Autodesk Fusion 360 part; units mm, degrees
note: some values were not read from the file. Set by a fixed rule: which face or edge a step refers to.
(part 2 of 4)
  spline S17 degree 5 poles (16.9837, -27.7093) (16.9833, -27.6954) (16.9825, -27.6677) (16.9812, -27.6262) (16.9792, -27.5708) (16.9764, -27.5018) (16.9734, -27.4329) (16.97, -27.364) (16.9664, -27.2952) (16.9624, -27.2266) (16.9582, -27.158) (16.9536, -27.0896) (16.9488, -27.0213) (16.9436, -26.953) (16.9381, -26.8849) (16.9323, -26.8169) (16.9262, -26.749) (16.9198, -26.6812) (16.9131, -26.6136) (16.906, -26.546) (16.8987, -26.4786) (16.891, -26.4113) (16.883, -26.3441) (16.8746, -26.2771) (16.866, -26.2101) (16.857, -26.1433) (16.8477, -26.0767) (16.838, -26.0102) (16.8281, -25.9438) (16.8178, -25.8775) (16.8071, -25.8114) (16.7961, -25.7455) (16.7848, -25.6797) (16.7731, -25.614) (16.761, -25.5485) (16.7486, -25.4831) (16.7359, -25.4179) (16.7228, -25.3529) (16.7093, -25.288) (16.6955, -25.2233) (16.6813, -25.1588) (16.6667, -25.0945) (16.6517, -25.0303) (16.6364, -24.9663) (16.6206, -24.9025) (16.6045, -24.8389) (16.5879, -24.7755) (16.571, -24.7123) (16.5537, -24.6492) (16.536, -24.5864) (16.5178, -24.5238) (16.4992, -24.4614) (16.4801, -24.3993) (16.4606, -24.3375) (16.4405, -24.2758) (16.4201, -24.2144) (16.3992, -24.1533) (16.3779, -24.0923) (16.3562, -24.0316) (16.3339, -23.9712) (16.3111, -23.9111) (16.2876, -23.8514) (16.2633, -23.7922) (16.2383, -23.7333) (16.2126, -23.6749) (16.1864, -23.6167) (16.1599, -23.5588) (16.1331, -23.501) (16.1057, -23.4436) (16.0774, -23.3868) (16.0476, -23.3309) (16.0221, -23.2873) (16.0018, -23.2552) (15.9877, -23.2342) (15.9805, -23.2237) knots -1 -1 -1 -1 -1 -1 -0.98571429 -0.97142857 -0.95714286 -0.94285714 -0.92857143 -0.91428571 -0.9 -0.88571429 -0.87142857 -0.85714286 -0.84285714 -0.82857143 -0.81428571 -0.8 -0.78571429 -0.77142857 -0.75714286 -0.74285714 -0.72857143 -0.71428571 -0.7 -0.68571429 -0.67142857 -0.65714286 -0.64285714 -0.62857143 -0.61428571 -0.6 -0.58571429 -0.57142857 -0.55714286 -0.54285714 -0.52857143 -0.51428571 -0.5 -0.48571429 -0.47142857 -0.45714286 -0.44285714 -0.42857143 -0.41428571 -0.4 -0.38571429 -0.37142857 -0.35714286 -0.34285714 -0.32857143 -0.31428571 -0.3 -0.28571429 -0.27142857 -0.25714286 -0.24285714 -0.22857143 -0.21428571 -0.2 -0.18571429 -0.17142857 -0.15714286 -0.14285714 -0.12857143 -0.11428571 -0.1 -0.08571429 -0.07142857 -0.05714286 -0.04285714 -0.02857143 -0.01428571 0 0 0 0 0 0
  line L17 (15.9805, -23.2237) -> (15.7785, -22.9298)
  arc A35 (15.9864, -21.6955) -> (15.7785, -22.9298) centre (16.5203, -22.42) ccw
  arc A36 (15.9864, -21.6955) -> (16.8187, -21.0569) centre (0, 0) ccw
  arc A37 (18.0647, -21.1755) -> (16.8187, -21.0569) centre (17.3803, -21.7601) ccw
  line L18 (18.0647, -21.1755) -> (18.2963, -21.4468)
  spline S18 degree 5 poles (18.2963, -21.4468) (18.3046, -21.4564) (18.3212, -21.4754) (18.3469, -21.5033) (18.3825, -21.5393) (18.4288, -21.5826) (18.4763, -21.6246) (18.5247, -21.6659) (18.5735, -21.7068) (18.6226, -21.7474) (18.6721, -21.7877) (18.7219, -21.8276) (18.7722, -21.867) (18.8232, -21.9058) (18.8747, -21.944) (18.9269, -21.9816) (18.9795, -22.0187) (19.0325, -22.0554) (19.0858, -22.0917) (19.1395, -22.1277) (19.1935, -22.1634) (19.2479, -22.1987) (19.3026, -22.2336) (19.3576, -22.2681) (19.413, -22.3022) (19.4688, -22.336) (19.5249, -22.3694) (19.5813, -22.4024) (19.638, -22.4351) (19.695, -22.4675) (19.7522, -22.4995) (19.8098, -22.5312) (19.8676, -22.5626) (19.9257, -22.5937) (19.9841, -22.6244) (20.0428, -22.6549) (20.1017, -22.685) (20.1609, -22.7148) (20.2203, -22.7443) (20.28, -22.7735) (20.3399, -22.8023) (20.4, -22.8309) (20.4604, -22.8592) (20.5211, -22.8872) (20.5819, -22.9149) (20.643, -22.9423) (20.7043, -22.9694) (20.7659, -22.9962) (20.8276, -23.0228) (20.8896, -23.049) (20.9518, -23.075) (21.0142, -23.1007) (21.0768, -23.1261) (21.1396, -23.1512) (21.2027, -23.176) (21.2659, -23.2006) (21.3293, -23.2249) (21.3929, -23.2489) (21.4567, -23.2726) (21.5207, -23.2961) (21.5849, -23.3193) (21.6493, -23.3422) (21.7139, -23.3649) (21.7786, -23.3872) (21.8436, -23.4094) (21.9087, -23.4312) (21.974, -23.4528) (22.0394, -23.4741) (22.1051, -23.4952) (22.1709, -23.516) (22.2369, -23.5365) (22.2898, -23.5527) (22.3295, -23.5648) (22.3561, -23.5727) (22.3694, -23.5767) knots 0 0 0 0 0 0 0.01428571 0.02857143 0.04285714 0.05714286 0.07142857 0.08571429 0.1 0.11428571 0.12857143 0.14285714 0.15714286 0.17142857 0.18571429 0.2 0.21428571 0.22857143 0.24285714 0.25714286 0.27142857 0.28571429 0.3 0.31428571 0.32857143 0.34285714 0.35714286 0.37142857 0.38571429 0.4 0.41428571 0.42857143 0.44285714 0.45714286 0.47142857 0.48571429 0.5 0.51428571 0.52857143 0.54285714 0.55714286 0.57142857 0.58571429 0.6 0.61428571 0.62857143 0.64285714 0.65714286 0.67142857 0.68571429 0.7 0.71428571 0.72857143 0.74285714 0.75714286 0.77142857 0.78571429 0.8 0.81428571 0.82857143 0.84285714 0.85714286 0.87142857 0.88571429 0.9 0.91428571 0.92857143 0.94285714 0.95714286 0.97142857 0.98571429 1 1 1 1 1 1
  arc A38 (22.3694, -23.5767) -> (23.5767, -22.3694) centre (0, 0) ccw
  spline S19 degree 5 poles (23.5767, -22.3694) (23.5727, -22.3561) (23.5648, -22.3295) (23.5527, -22.2898) (23.5365, -22.2369) (23.516, -22.1709) (23.4952, -22.1051) (23.4741, -22.0394) (23.4528, -21.974) (23.4312, -21.9087) (23.4094, -21.8436) (23.3872, -21.7786) (23.3649, -21.7139) (23.3422, -21.6493) (23.3193, -21.5849) (23.2961, -21.5207) (23.2726, -21.4567) (23.2489, -21.3929) (23.2249, -21.3293) (23.2006, -21.2659) (23.176, -21.2027) (23.1512, -21.1396) (23.1261, -21.0768) (23.1007, -21.0142) (23.075, -20.9518) (23.049, -20.8896) (23.0228, -20.8276) (22.9962, -20.7659) (22.9694, -20.7043) (22.9423, -20.643) (22.9149, -20.5819) (22.8872, -20.5211) (22.8592, -20.4604) (22.8309, -20.4) (22.8023, -20.3399) (22.7735, -20.28) (22.7443, -20.2203) (22.7148, -20.1609) (22.685, -20.1017) (22.6549, -20.0428) (22.6244, -19.9841) (22.5937, -19.9257) (22.5626, -19.8676) (22.5312, -19.8098) (22.4995, -19.7522) (22.4675, -19.695) (22.4351, -19.638) (22.4024, -19.5813) (22.3694, -19.5249) (22.336, -19.4688) (22.3022, -19.413) (22.2681, -19.3576) (22.2336, -19.3026) (22.1987, -19.2479) (22.1634, -19.1935) (22.1277, -19.1395) (22.0917, -19.0858) (22.0554, -19.0325) (22.0187, -18.9795) (21.9816, -18.9269) (21.944, -18.8747) (21.9058, -18.8232) (21.867, -18.7722) (21.8276, -18.7219) (21.7877, -18.6721) (21.7474, -18.6226) (21.7068, -18.5735) (21.6659, -18.5247) (21.6246, -18.4763) (21.5826, -18.4288) (21.5393, -18.3825) (21.5033, -18.3469) (21.4754, -18.3212) (21.4564, -18.3046) (21.4468, -18.2963) knots -1 -1 -1 -1 -1 -1 -0.98571429 -0.97142857 -0.95714286 -0.94285714 -0.92857143 -0.91428571 -0.9 -0.88571429 -0.87142857 -0.85714286 -0.84285714 -0.82857143 -0.81428571 -0.8 -0.78571429 -0.77142857 -0.75714286 -0.74285714 -0.72857143 -0.71428571 -0.7 -0.68571429 -0.67142857 -0.65714286 -0.64285714 -0.62857143 -0.61428571 -0.6 -0.58571429 -0.57142857 -0.55714286 -0.54285714 -0.52857143 -0.51428571 -0.5 -0.48571429 -0.47142857 -0.45714286 -0.44285714 -0.42857143 -0.41428571 -0.4 -0.38571429 -0.37142857 -0.35714286 -0.34285714 -0.32857143 -0.31428571 -0.3 -0.28571429 -0.27142857 -0.25714286 -0.24285714 -0.22857143 -0.21428571 -0.2 -0.18571429 -0.17142857 -0.15714286 -0.14285714 -0.12857143 -0.11428571 -0.1 -0.08571429 -0.07142857 -0.05714286 -0.04285714 -0.02857143 -0.01428571 0 0 0 0 0 0
  line L19 (21.4468, -18.2963) -> (21.1755, -18.0647)
  arc A39 (21.0569, -16.8187) -> (21.1755, -18.0647) centre (21.7601, -17.3803) ccw
  arc A40 (21.0569, -16.8187) -> (21.6955, -15.9864) centre (0, 0) ccw
  arc A41 (22.9298, -15.7785) -> (21.6955, -15.9864) centre (22.42, -16.5203) ccw
  line L20 (22.9298, -15.7785) -> (23.2237, -15.9805)
  spline S20 degree 5 poles (23.2237, -15.9805) (23.2342, -15.9877) (23.2552, -16.0018) (23.2873, -16.0221) (23.3309, -16.0476) (23.3868, -16.0774) (23.4436, -16.1057) (23.501, -16.1331) (23.5588, -16.1599) (23.6167, -16.1864) (23.6749, -16.2126) (23.7333, -16.2383) (23.7922, -16.2633) (23.8514, -16.2876) (23.9111, -16.3111) (23.9712, -16.3339) (24.0316, -16.3562) (24.0923, -16.3779) (24.1533, -16.3992) (24.2144, -16.4201) (24.2758, -16.4405) (24.3375, -16.4606) (24.3993, -16.4801) (24.4614, -16.4992) (24.5238, -16.5178) (24.5864, -16.536) (24.6492, -16.5537) (24.7123, -16.571) (24.7755, -16.5879) (24.8389, -16.6045) (24.9025, -16.6206) (24.9663, -16.6364) (25.0303, -16.6517) (25.0945, -16.6667) (25.1588, -16.6813) (25.2233, -16.6955) (25.288, -16.7093) (25.3529, -16.7228) (25.4179, -16.7359) (25.4831, -16.7486) (25.5485, -16.761) (25.614, -16.7731) (25.6797, -16.7848) (25.7455, -16.7961) (25.8114, -16.8071) (25.8775, -16.8178) (25.9438, -16.8281) (26.0102, -16.838) (26.0767, -16.8477) (26.1433, -16.857) (26.2101, -16.866) (26.2771, -16.8746) (26.3441, -16.883) (26.4113, -16.891) (26.4786, -16.8987) (26.546, -16.906) (26.6136, -16.9131) (26.6812, -16.9198) (26.749, -16.9262) (26.8169, -16.9323) (26.8849, -16.9381) (26.953, -16.9436) (27.0213, -16.9488) (27.0896, -16.9536) (27.158, -16.9582) (27.2266, -16.9624) (27.2952, -16.9664) (27.364, -16.97) (27.4329, -16.9734) (27.5018, -16.9764) (27.5708, -16.9792) (27.6262, -16.9812) (27.6677, -16.9825) (27.6954, -16.9833) (27.7093, -16.9837) knots 0 0 0 0 0 0 0.01428571 0.02857143 0.04285714 0.05714286 0.07142857 0.08571429 0.1 0.11428571 0.12857143 0.14285714 0.15714286 0.17142857 0.18571429 0.2 0.21428571 0.22857143 0.24285714 0.25714286 0.27142857 0.28571429 0.3 0.31428571 0.32857143 0.34285714 0.35714286 0.37142857 0.38571429 0.4 0.41428571 0.42857143 0.44285714 0.45714286 0.47142857 0.48571429 0.5 0.51428571 0.52857143 0.54285714 0.55714286 0.57142857 0.58571429 0.6 0.61428571 0.62857143 0.64285714 0.65714286 0.67142857 0.68571429 0.7 0.71428571 0.72857143 0.74285714 0.75714286 0.77142857 0.78571429 0.8 0.81428571 0.82857143 0.84285714 0.85714286 0.87142857 0.88571429 0.9 0.91428571 0.92857143 0.94285714 0.95714286 0.97142857 0.98571429 1 1 1 1 1 1
  arc A42 (27.7093, -16.9837) -> (28.563, -15.5051) centre (0, 0) ccw
  spline S21 degree 5 poles (28.563, -15.5051) (28.5557, -15.4933) (28.5411, -15.4697) (28.5192, -15.4344) (28.4898, -15.3875) (28.4529, -15.329) (28.4158, -15.2709) (28.3785, -15.2129) (28.3409, -15.1552) (28.3032, -15.0977) (28.2652, -15.0405) (28.2271, -14.9835) (28.1887, -14.9267) (28.1501, -14.8702) (28.1113, -14.814) (28.0723, -14.758) (28.033, -14.7022) (27.9936, -14.6467) (27.9539, -14.5915) (27.9141, -14.5365) (27.874, -14.4818) (27.8337, -14.4274) (27.7931, -14.3732) (27.7524, -14.3193) (27.7114, -14.2657) (27.6703, -14.2123) (27.6289, -14.1592) (27.5873, -14.1064) (27.5454, -14.0539) (27.5034, -14.0017) (27.4611, -13.9498) (27.4186, -13.8982) (27.3759, -13.8469) (27.3329, -13.7958) (27.2897, -13.7451) (27.2463, -13.6947) (27.2027, -13.6446) (27.1588, -13.5949) (27.1147, -13.5454) (27.0704, -13.4963) (27.0258, -13.4475) (26.981, -13.3991) (26.936, -13.351) (26.8907, -13.3033) (26.8451, -13.2559) (26.7993, -13.2089) (26.7533, -13.1622) (26.7071, -13.1159) (26.6606, -13.07) (26.6138, -13.0245) (26.5668, -12.9793) (26.5195, -12.9346) (26.4719, -12.8904) (26.424, -12.8466) (26.3758, -12.8032) (26.3274, -12.7603) (26.2788, -12.7178) (26.2299, -12.6756) (26.1807, -12.6339) (26.1312, -12.5927) (26.0814, -12.5521) (26.0312, -12.5122) (25.9805, -12.473) (25.9294, -12.4346) (25.878, -12.3968) (25.8262, -12.3595) (25.7743, -12.3225) (25.7222, -12.2859) (25.6698, -12.2499) (25.6169, -12.2149) (25.5631, -12.1814) (25.5192, -12.1563) (25.4856, -12.1387) (25.4629, -12.1275) (25.4514, -12.1221) knots -1 -1 -1 -1 -1 -1 -0.98571429 -0.97142857 -0.95714286 -0.94285714 -0.92857143 -0.91428571 -0.9 -0.88571429 -0.87142857 -0.85714286 -0.84285714 -0.82857143 -0.81428571 -0.8 -0.78571429 -0.77142857 -0.75714286 -0.74285714 -0.72857143 -0.71428571 -0.7 -0.68571429 -0.67142857 -0.65714286 -0.64285714 -0.62857143 -0.61428571 -0.6 -0.58571429 -0.57142857 -0.55714286 -0.54285714 -0.52857143 -0.51428571 -0.5 -0.48571429 -0.47142857 -0.45714286 -0.44285714 -0.42857143 -0.41428571 -0.4 -0.38571429 -0.37142857 -0.35714286 -0.34285714 -0.32857143 -0.31428571 -0.3 -0.28571429 -0.27142857 -0.25714286 -0.24285714 -0.22857143 -0.21428571 -0.2 -0.18571429 -0.17142857 -0.15714286 -0.14285714 -0.12857143 -0.11428571 -0.1 -0.08571429 -0.07142857 -0.05714286 -0.04285714 -0.02857143 -0.01428571 0 0 0 0 0 0
  line L21 (25.4514, -12.1221) -> (25.1295, -11.9685)
  arc A43 (24.6924, -10.7957) -> (25.1295, -11.9685) centre (25.517, -11.1562) ccw
  arc A44 (24.6924, -10.7957) -> (25.0938, -9.8265) centre (0, 0) ccw
  arc A45 (26.2322, -9.3062) -> (25.0938, -9.8265) centre (25.9319, -10.1546) ccw
  line L22 (26.2322, -9.3062) -> (26.5685, -9.4253)
  spline S22 degree 5 poles (26.5685, -9.4253) (26.5804, -9.4295) (26.6044, -9.4376) (26.6406, -9.449) (26.6894, -9.4623) (26.7511, -9.4767) (26.8133, -9.4893) (26.8758, -9.5009) (26.9385, -9.5119) (27.0014, -9.5225) (27.0643, -9.5326) (27.1274, -9.5423) (27.1907, -9.5513) (27.2542, -9.5594) (27.318, -9.5667) (27.3819, -9.5732) (27.4461, -9.579) (27.5103, -9.5843) (27.5747, -9.5891) (27.6392, -9.5934) (27.7038, -9.5973) (27.7685, -9.6007) (27.8333, -9.6036) (27.8982, -9.6059) (27.9633, -9.6078) (28.0285, -9.6091) (28.0937, -9.61) (28.1591, -9.6104) (28.2246, -9.6104) (28.2901, -9.6099) (28.3557, -9.609) (28.4214, -9.6077) (28.4872, -9.606) (28.553, -9.6039) (28.619, -9.6013) (28.685, -9.5983) (28.7511, -9.5949) (28.8172, -9.5911) (28.8834, -9.587) (28.9497, -9.5824) (29.016, -9.5775) (29.0824, -9.5721) (29.1489, -9.5664) (29.2154, -9.5604) (29.2819, -9.5539) (29.3485, -9.5471) (29.4152, -9.5399) (29.4819, -9.5324) (29.5487, -9.5245) (29.6154, -9.5162) (29.6823, -9.5076) (29.7492, -9.4986) (29.8161, -9.4893) (29.8831, -9.4797) (29.9501, -9.4697) (30.0171, -9.4594) (30.0842, -9.4487) (30.1513, -9.4377) (30.2184, -9.4263) (30.2855, -9.4146) (30.3527, -9.4026) (30.42, -9.3903) (30.4872, -9.3776) (30.5545, -9.3646) (30.6218, -9.3513) (30.6891, -9.3377) (30.7564, -9.3237) (30.8238, -9.3095) (30.8911, -9.2949) (30.9585, -9.28) (31.0259, -9.2648) (31.0799, -9.2524) (31.1203, -9.2429) (31.1473, -9.2365) (31.1608, -9.2333) knots 0 0 0 0 0 0 0.01428571 0.02857143 0.04285714 0.05714286 0.07142857 0.08571429 0.1 0.11428571 0.12857143 0.14285714 0.15714286 0.17142857 0.18571429 0.2 0.21428571 0.22857143 0.24285714 0.25714286 0.27142857 0.28571429 0.3 0.31428571 0.32857143 0.34285714 0.35714286 0.37142857 0.38571429 0.4 0.41428571 0.42857143 0.44285714 0.45714286 0.47142857 0.48571429 0.5 0.51428571 0.52857143 0.54285714 0.55714286 0.57142857 0.58571429 0.6 0.61428571 0.62857143 0.64285714 0.65714286 0.67142857 0.68571429 0.7 0.71428571 0.72857143 0.74285714 0.75714286 0.77142857 0.78571429 0.8 0.81428571 0.82857143 0.84285714 0.85714286 0.87142857 0.88571429 0.9 0.91428571 0.92857143 0.94285714 0.95714286 0.97142857 0.98571429 1 1 1 1 1 1
  arc A46 (31.1608, -9.2333) -> (31.6027, -7.5841) centre (0, 0) ccw
  spline S23 degree 5 poles (31.6027, -7.5841) (31.5926, -7.5746) (31.5725, -7.5556) (31.5421, -7.5272) (31.5016, -7.4894) (31.4509, -7.4426) (31.4, -7.396) (31.3489, -7.3496) (31.2977, -7.3036) (31.2464, -7.2579) (31.1949, -7.2124) (31.1433, -7.1672) (31.0915, -7.1223) (31.0396, -7.0777) (30.9876, -7.0335) (30.9354, -6.9895) (30.883, -6.9458) (30.8306, -6.9024) (30.778, -6.8593) (30.7252, -6.8165) (30.6724, -6.774) (30.6193, -6.7319) (30.5662, -6.69) (30.5129, -6.6485) (30.4594, -6.6073) (30.4058, -6.5664) (30.3521, -6.5259) (30.2983, -6.4857) (30.2443, -6.4458) (30.1901, -6.4062) (30.1358, -6.367) (30.0814, -6.3282) (30.0269, -6.2896) (29.9722, -6.2515) (29.9173, -6.2137) (29.8624, -6.1762) (29.8073, -6.1391) (29.752, -6.1024) (29.6966, -6.0661) (29.6411, -6.0301) (29.5854, -5.9945) (29.5296, -5.9593) (29.4736, -5.9245) (29.4175, -5.8902) (29.3613, -5.8562) (29.3049, -5.8226) (29.2484, -5.7895) (29.1917, -5.7567) (29.1349, -5.7244) (29.0779, -5.6925) (29.0208, -5.6611) (28.9636, -5.6301) (28.9061, -5.5997) (28.8486, -5.5698) (28.7908, -5.5404) (28.7329, -5.5114) (28.6749, -5.483) (28.6168, -5.4549) (28.5585, -5.4274) (28.5, -5.4004) (28.4414, -5.374) (28.3826, -5.3485) (28.3235, -5.3237) (28.2642, -5.2998) (28.2047, -5.2766) (28.1451, -5.254) (28.0854, -5.2318) (28.0256, -5.2099) (27.9656, -5.1887) (27.9054, -5.1685) (27.8448, -5.1501) (27.7959, -5.1373) (27.7589, -5.1289) (27.7341, -5.124) (27.7216, -5.1217) knots -1 -1 -1 -1 -1 -1 -0.98571429 -0.97142857 -0.95714286 -0.94285714 -0.92857143 -0.91428571 -0.9 -0.88571429 -0.87142857 -0.85714286 -0.84285714 -0.82857143 -0.81428571 -0.8 -0.78571429 -0.77142857 -0.75714286 -0.74285714 -0.72857143 -0.71428571 -0.7 -0.68571429 -0.67142857 -0.65714286 -0.64285714 -0.62857143 -0.61428571 -0.6 -0.58571429 -0.57142857 -0.55714286 -0.54285714 -0.52857143 -0.51428571 -0.5 -0.48571429 -0.47142857 -0.45714286 -0.44285714 -0.42857143 -0.41428571 -0.4 -0.38571429 -0.37142857 -0.35714286 -0.34285714 -0.32857143 -0.31428571 -0.3 -0.28571429 -0.27142857 -0.25714286 -0.24285714 -0.22857143 -0.21428571 -0.2 -0.18571429 -0.17142857 -0.15714286 -0.14285714 -0.12857143 -0.11428571 -0.1 -0.08571429 -0.07142857 -0.05714286 -0.04285714 -0.02857143 -0.01428571 0 0 0 0 0 0
  line L23 (27.7216, -5.1217) -> (27.3709, -5.0567)
  arc A47 (26.6451, -4.037) -> (27.3709, -5.0567) centre (27.535, -4.1718) ccw
  arc A48 (26.6451, -4.037) -> (26.782, -2.9969) centre (0, 0) ccw
  arc A49 (27.747, -2.1997) -> (26.782, -2.9969) centre (27.6765, -3.097) ccw
  line L24 (27.747, -2.1997) -> (28.1026, -2.2277)
  spline S24 degree 5 poles (28.1026, -2.2277) (28.1152, -2.2287) (28.1405, -2.2303) (28.1784, -2.2319) (28.229, -2.2322) (28.2923, -2.2301) (28.3557, -2.2262) (28.419, -2.2212) (28.4825, -2.2155) (28.5459, -2.2095) (28.6093, -2.2031) (28.6728, -2.1961) (28.7363, -2.1883) (28.7997, -2.1797) (28.8632, -2.1703) (28.9266, -2.16) (28.9901, -2.1491) (29.0535, -2.1375) (29.117, -2.1255) (29.1804, -2.113) (29.2438, -2.1) (29.3071, -2.0865) (29.3705, -2.0726) (29.4338, -2.058) (29.4972, -2.043) (29.5604, -2.0274) (29.6237, -2.0113) (29.687, -1.9948) (29.7502, -1.9778) (29.8134, -1.9604) (29.8765, -1.9426) (29.9396, -1.9244) (30.0027, -1.9057) (30.0658, -1.8865) (30.1288, -1.867) (30.1918, -1.847) (30.2547, -1.8267) (30.3177, -1.8059) (30.3805, -1.7847) (30.4434, -1.7632) (30.5062, -1.7412) (30.5689, -1.7189) (30.6316, -1.6962) (30.6943, -1.6731) (30.7569, -1.6497) (30.8195, -1.6258) (30.882, -1.6016) (30.9445, -1.5771) (31.0069, -1.5522) (31.0693, -1.5269) (31.1316, -1.5013) (31.1939, -1.4753) (31.2562, -1.449) (31.3183, -1.4224) (31.3805, -1.3954) (31.4425, -1.368) (31.5046, -1.3404) (31.5665, -1.3124) (31.6284, -1.284) (31.6903, -1.2554) (31.7521, -1.2264) (31.8138, -1.1971) (31.8755, -1.1674) (31.9371, -1.1375) (31.9986, -1.1072) (32.0601, -1.0766) (32.1216, -1.0457) (32.1829, -1.0145) (32.2442, -0.983) (32.3055, -0.9511) (32.3666, -0.919) (32.4155, -0.893) (32.4522, -0.8734) (32.4766, -0.8603) (32.4888, -0.8537) knots 0 0 0 0 0 0 0.01428571 0.02857143 0.04285714 0.05714286 0.07142857 0.08571429 0.1 0.11428571 0.12857143 0.14285714 0.15714286 0.17142857 0.18571429 0.2 0.21428571 0.22857143 0.24285714 0.25714286 0.27142857 0.28571429 0.3 0.31428571 0.32857143 0.34285714 0.35714286 0.37142857 0.38571429 0.4 0.41428571 0.42857143 0.44285714 0.45714286 0.47142857 0.48571429 0.5 0.51428571 0.52857143 0.54285714 0.55714286 0.57142857 0.58571429 0.6 0.61428571 0.62857143 0.64285714 0.65714286 0.67142857 0.68571429 0.7 0.71428571 0.72857143 0.74285714 0.75714286 0.77142857 0.78571429 0.8 0.81428571 0.82857143 0.84285714 0.85714286 0.87142857 0.88571429 0.9 0.91428571 0.92857143 0.94285714 0.95714286 0.97142857 0.98571429 1 1 1 1 1 1
  arc A50 (32.4888, -0.8537) -> (32.4888, 0.8537) centre (0, 0) ccw
  spline S25 degree 5 poles (32.4888, 0.8537) (32.4766, 0.8603) (32.4522, 0.8734) (32.4155, 0.893) (32.3666, 0.919) (32.3055, 0.9511) (32.2442, 0.983) (32.1829, 1.0145) (32.1216, 1.0457) (32.0601, 1.0766) (31.9986, 1.1072) (31.9371, 1.1375) (31.8755, 1.1674) (31.8138, 1.1971) (31.7521, 1.2264) (31.6903, 1.2554) (31.6284, 1.284) (31.5665, 1.3124) (31.5046, 1.3404) (31.4425, 1.368) (31.3805, 1.3954) (31.3183, 1.4224) (31.2562, 1.449) (31.1939, 1.4753) (31.1316, 1.5013) (31.0693, 1.5269) (31.0069, 1.5522) (30.9445, 1.5771) (30.882, 1.6016) (30.8195, 1.6258) (30.7569, 1.6497) (30.6943, 1.6731) (30.6316, 1.6962) (30.5689, 1.7189) (30.5062, 1.7412) (30.4434, 1.7632) (30.3805, 1.7847) (30.3177, 1.8059) (30.2547, 1.8267) (30.1918, 1.847) (30.1288, 1.867) (30.0658, 1.8865) (30.0027, 1.9057) (29.9396, 1.9244) (29.8765, 1.9426) (29.8134, 1.9604) (29.7502, 1.9778) (29.687, 1.9948) (29.6237, 2.0113) (29.5604, 2.0274) (29.4972, 2.043) (29.4338, 2.058) (29.3705, 2.0726) (29.3071, 2.0865) (29.2438, 2.1) (29.1804, 2.113) (29.117, 2.1255) (29.0535, 2.1375) (28.9901, 2.1491) (28.9266, 2.16) (28.8632, 2.1703) (28.7997, 2.1797) (28.7363, 2.1883) (28.6728, 2.1961) (28.6093, 2.2031) (28.5459, 2.2095) (28.4825, 2.2155) (28.419, 2.2212) (28.3557, 2.2262) (28.2923, 2.2301) (28.229, 2.2322) (28.1784, 2.2319) (28.1405, 2.2303) (28.1152, 2.2287) (28.1026, 2.2277) knots -1 -1 -1 -1 -1 -1 -0.98571429 -0.97142857 -0.95714286 -0.94285714 -0.92857143 -0.91428571 -0.9 -0.88571429 -0.87142857 -0.85714286 -0.84285714 -0.82857143 -0.81428571 -0.8 -0.78571429 -0.77142857 -0.75714286 -0.74285714 -0.72857143 -0.71428571 -0.7 -0.68571429 -0.67142857 -0.65714286 -0.64285714 -0.62857143 -0.61428571 -0.6 -0.58571429 -0.57142857 -0.55714286 -0.54285714 -0.52857143 -0.51428571 -0.5 -0.48571429 -0.47142857 -0.45714286 -0.44285714 -0.42857143 -0.41428571 -0.4 -0.38571429 -0.37142857 -0.35714286 -0.34285714 -0.32857143 -0.31428571 -0.3 -0.28571429 -0.27142857 -0.25714286 -0.24285714 -0.22857143 -0.21428571 -0.2 -0.18571429 -0.17142857 -0.15714286 -0.14285714 -0.12857143 -0.11428571 -0.1 -0.08571429 -0.07142857 -0.05714286 -0.04285714 -0.02857143 -0.01428571 0 0 0 0 0 0
  line L25 (28.1026, 2.2277) -> (27.747, 2.1997)
  arc A51 (26.782, 2.9969) -> (27.747, 2.1997) centre (27.6765, 3.097) ccw
  arc A52 (26.782, 2.9969) -> (26.6451, 4.037) centre (0, 0) ccw
  arc A53 (27.3709, 5.0567) -> (26.6451, 4.037) centre (27.535, 4.1718) ccw
  line L26 (27.3709, 5.0567) -> (27.7216, 5.1217)
  spline S26 degree 5 poles (27.7216, 5.1217) (27.7341, 5.124) (27.7589, 5.1289) (27.7959, 5.1373) (27.8448, 5.1501) (27.9054, 5.1685) (27.9656, 5.1887) (28.0256, 5.2099) (28.0854, 5.2318) (28.1451, 5.254) (28.2047, 5.2766) (28.2642, 5.2998) (28.3235, 5.3237) (28.3826, 5.3485) (28.4414, 5.374) (28.5, 5.4004) (28.5585, 5.4274) (28.6168, 5.4549) (28.6749, 5.483) (28.7329, 5.5114) (28.7908, 5.5404) (28.8486, 5.5698) (28.9061, 5.5997) (28.9636, 5.6301) (29.0208, 5.6611) (29.0779, 5.6925) (29.1349, 5.7244) (29.1917, 5.7567) (29.2484, 5.7895) (29.3049, 5.8226) (29.3613, 5.8562) (29.4175, 5.8902) (29.4736, 5.9245) (29.5296, 5.9593) (29.5854, 5.9945) (29.6411, 6.0301) (29.6966, 6.0661) (29.752, 6.1024) (29.8073, 6.1391) (29.8624, 6.1762) (29.9173, 6.2137) (29.9722, 6.2515) (30.0269, 6.2896) (30.0814, 6.3282) (30.1358, 6.367) (30.1901, 6.4062) (30.2443, 6.4458) (30.2983, 6.4857) (30.3521, 6.5259) (30.4058, 6.5664) (30.4594, 6.6073) (30.5129, 6.6485) (30.5662, 6.69) (30.6193, 6.7319) (30.6724, 6.774) (30.7252, 6.8165) (30.778, 6.8593) (30.8306, 6.9024) (30.883, 6.9458) (30.9354, 6.9895) (30.9876, 7.0335) (31.0396, 7.0777) (31.0915, 7.1223) (31.1433, 7.1672) (31.1949, 7.2124) (31.2464, 7.2579) (31.2977, 7.3036) (31.3489, 7.3496) (31.4, 7.396) (31.4509, 7.4426) (31.5016, 7.4894) (31.5421, 7.5272) (31.5725, 7.5556) (31.5926, 7.5746) (31.6027, 7.5841) knots 0 0 0 0 0 0 0.01428571 0.02857143 0.04285714 0.05714286 0.07142857 0.08571429 0.1 0.11428571 0.12857143 0.14285714 0.15714286 0.17142857 0.18571429 0.2 0.21428571 0.22857143 0.24285714 0.25714286 0.27142857 0.28571429 0.3 0.31428571 0.32857143 0.34285714 0.35714286 0.37142857 0.38571429 0.4 0.41428571 0.42857143 0.44285714 0.45714286 0.47142857 0.48571429 0.5 0.51428571 0.52857143 0.54285714 0.55714286 0.57142857 0.58571429 0.6 0.61428571 0.62857143 0.64285714 0.65714286 0.67142857 0.68571429 0.7 0.71428571 0.72857143 0.74285714 0.75714286 0.77142857 0.78571429 0.8 0.81428571 0.82857143 0.84285714 0.85714286 0.87142857 0.88571429 0.9 0.91428571 0.92857143 0.94285714 0.95714286 0.97142857 0.98571429 1 1 1 1 1 1
  arc A54 (31.6027, 7.5841) -> (31.1608, 9.2333) centre (0, 0) ccw
  spline S27 degree 5 poles (31.1608, 9.2333) (31.1473, 9.2365) (31.1203, 9.2429) (31.0799, 9.2524) (31.0259, 9.2648) (30.9585, 9.28) (30.8911, 9.2949) (30.8238, 9.3095) (30.7564, 9.3237) (30.6891, 9.3377) (30.6218, 9.3513) (30.5545, 9.3646) (30.4872, 9.3776) (30.42, 9.3903) (30.3527, 9.4026) (30.2855, 9.4146) (30.2184, 9.4263) (30.1513, 9.4377) (30.0842, 9.4487) (30.0171, 9.4594) (29.9501, 9.4697) (29.8831, 9.4797) (29.8161, 9.4893) (29.7492, 9.4986) (29.6823, 9.5076) (29.6154, 9.5162) (29.5487, 9.5245) (29.4819, 9.5324) (29.4152, 9.5399) (29.3485, 9.5471) (29.2819, 9.5539) (29.2154, 9.5604) (29.1489, 9.5664) (29.0824, 9.5721) (29.016, 9.5775) (28.9497, 9.5824) (28.8834, 9.587) (28.8172, 9.5911) (28.7511, 9.5949) (28.685, 9.5983) (28.619, 9.6013) (28.553, 9.6039) (28.4872, 9.606) (28.4214, 9.6077) (28.3557, 9.609) (28.2901, 9.6099) (28.2246, 9.6104) (28.1591, 9.6104) (28.0937, 9.61) (28.0285, 9.6091) (27.9633, 9.6078) (27.8982, 9.6059) (27.8333, 9.6036) (27.7685, 9.6007) (27.7038, 9.5973) (27.6392, 9.5934) (27.5747, 9.5891) (27.5103, 9.5843) (27.4461, 9.579) (27.3819, 9.5732) (27.318, 9.5667) (27.2542, 9.5594) (27.1907, 9.5513) (27.1274, 9.5423) (27.0643, 9.5326) (27.0014, 9.5225) (26.9385, 9.5119) (26.8758, 9.5009) (26.8133, 9.4893) (26.7511, 9.4767) (26.6894, 9.4623) (26.6406, 9.449) (26.6044, 9.4376) (26.5804, 9.4295) (26.5685, 9.4253) knots -1 -1 -1 -1 -1 -1 -0.98571429 -0.97142857 -0.95714286 -0.94285714 -0.92857143 -0.91428571 -0.9 -0.88571429 -0.87142857 -0.85714286 -0.84285714 -0.82857143 -0.81428571 -0.8 -0.78571429 -0.77142857 -0.75714286 -0.74285714 -0.72857143 -0.71428571 -0.7 -0.68571429 -0.67142857 -0.65714286 -0.64285714 -0.62857143 -0.61428571 -0.6 -0.58571429 -0.57142857 -0.55714286 -0.54285714 -0.52857143 -0.51428571 -0.5 -0.48571429 -0.47142857 -0.45714286 -0.44285714 -0.42857143 -0.41428571 -0.4 -0.38571429 -0.37142857 -0.35714286 -0.34285714 -0.32857143 -0.31428571 -0.3 -0.28571429 -0.27142857 -0.25714286 -0.24285714 -0.22857143 -0.21428571 -0.2 -0.18571429 -0.17142857 -0.15714286 -0.14285714 -0.12857143 -0.11428571 -0.1 -0.08571429 -0.07142857 -0.05714286 -0.04285714 -0.02857143 -0.01428571 0 0 0 0 0 0
  line L27 (26.5685, 9.4253) -> (26.2322, 9.3062)
  arc A55 (25.0938, 9.8265) -> (26.2322, 9.3062) centre (25.9319, 10.1546) ccw
  arc A56 (25.0938, 9.8265) -> (24.6924, 10.7957) centre (0, 0) ccw
  arc A57 (25.1295, 11.9685) -> (24.6924, 10.7957) centre (25.517, 11.1562) ccw
  line L28 (25.1295, 11.9685) -> (25.4514, 12.1221)
  spline S28 degree 5 poles (25.4514, 12.1221) (25.4629, 12.1275) (25.4856, 12.1387) (25.5192, 12.1563) (25.5631, 12.1814) (25.6169, 12.2149) (25.6698, 12.2499) (25.7222, 12.2859) (25.7743, 12.3225) (25.8262, 12.3595) (25.878, 12.3968) (25.9294, 12.4346) (25.9805, 12.473) (26.0312, 12.5122) (26.0814, 12.5521) (26.1312, 12.5927) (26.1807, 12.6339) (26.2299, 12.6756) (26.2788, 12.7178) (26.3274, 12.7603) (26.3758, 12.8032) (26.424, 12.8466) (26.4719, 12.8904) (26.5195, 12.9346) (26.5668, 12.9793) (26.6138, 13.0245) (26.6606, 13.07) (26.7071, 13.1159) (26.7533, 13.1622) (26.7993, 13.2089) (26.8451, 13.2559) (26.8907, 13.3033) (26.936, 13.351) (26.981, 13.3991) (27.0258, 13.4475) (27.0704, 13.4963) (27.1147, 13.5454) (27.1588, 13.5949) (27.2027, 13.6446) (27.2463, 13.6947) (27.2897, 13.7451) (27.3329, 13.7958) (27.3759, 13.8469) (27.4186, 13.8982) (27.4611, 13.9498) (27.5034, 14.0017) (27.5454, 14.0539) (27.5873, 14.1064) (27.6289, 14.1592) (27.6703, 14.2123) (27.7114, 14.2657) (27.7524, 14.3193) (27.7931, 14.3732) (27.8337, 14.4274) (27.874, 14.4818) (27.9141, 14.5365) (27.9539, 14.5915) (27.9936, 14.6467) (28.033, 14.7022) (28.0723, 14.758) (28.1113, 14.814) (28.1501, 14.8702) (28.1887, 14.9267) (28.2271, 14.9835) (28.2652, 15.0405) (28.3032, 15.0977) (28.3409, 15.1552) (28.3785, 15.2129) (28.4158, 15.2709) (28.4529, 15.329) (28.4898, 15.3875) (28.5192, 15.4344) (28.5411, 15.4697) (28.5557, 15.4933) (28.563, 15.5051) knots 0 0 0 0 0 0 0.01428571 0.02857143 0.04285714 0.05714286 0.07142857 0.08571429 0.1 0.11428571 0.12857143 0.14285714 0.15714286 0.17142857 0.18571429 0.2 0.21428571 0.22857143 0.24285714 0.25714286 0.27142857 0.28571429 0.3 0.31428571 0.32857143 0.34285714 0.35714286 0.37142857 0.38571429 0.4 0.41428571 0.42857143 0.44285714 0.45714286 0.47142857 0.48571429 0.5 0.51428571 0.52857143 0.54285714 0.55714286 0.57142857 0.58571429 0.6 0.61428571 0.62857143 0.64285714 0.65714286 0.67142857 0.68571429 0.7 0.71428571 0.72857143 0.74285714 0.75714286 0.77142857 0.78571429 0.8 0.81428571 0.82857143 0.84285714 0.85714286 0.87142857 0.88571429 0.9 0.91428571 0.92857143 0.94285714 0.95714286 0.97142857 0.98571429 1 1 1 1 1 1
  arc A58 (28.563, 15.5051) -> (27.7093, 16.9837) centre (0, 0) ccw
  spline S29 degree 5 poles (27.7093, 16.9837) (27.6954, 16.9833) (27.6677, 16.9825) (27.6262, 16.9812) (27.5708, 16.9792) (27.5018, 16.9764) (27.4329, 16.9734) (27.364, 16.97) (27.2952, 16.9664) (27.2266, 16.9624) (27.158, 16.9582) (27.0896, 16.9536) (27.0213, 16.9488) (26.953, 16.9436) (26.8849, 16.9381) (26.8169, 16.9323) (26.749, 16.9262) (26.6812, 16.9198) (26.6136, 16.9131) (26.546, 16.906) (26.4786, 16.8987) (26.4113, 16.891) (26.3441, 16.883) (26.2771, 16.8746) (26.2101, 16.866) (26.1433, 16.857) (26.0767, 16.8477) (26.0102, 16.838) (25.9438, 16.8281) (25.8775, 16.8178) (25.8114, 16.8071) (25.7455, 16.7961) (25.6797, 16.7848) (25.614, 16.7731) (25.5485, 16.761) (25.4831, 16.7486) (25.4179, 16.7359) (25.3529, 16.7228) (25.288, 16.7093) (25.2233, 16.6955) (25.1588, 16.6813) (25.0945, 16.6667) (25.0303, 16.6517) (24.9663, 16.6364) (24.9025, 16.6206) (24.8389, 16.6045) (24.7755, 16.5879) (24.7123, 16.571) (24.6492, 16.5537) (24.5864, 16.536) (24.5238, 16.5178) (24.4614, 16.4992) (24.3993, 16.4801) (24.3375, 16.4606) (24.2758, 16.4405) (24.2144, 16.4201) (24.1533, 16.3992) (24.0923, 16.3779) (24.0316, 16.3562) (23.9712, 16.3339) (23.9111, 16.3111) (23.8514, 16.2876) (23.7922, 16.2633) (23.7333, 16.2383) (23.6749, 16.2126) (23.6167, 16.1864) (23.5588, 16.1599) (23.501, 16.1331) (23.4436, 16.1057) (23.3868, 16.0774) (23.3309, 16.0476) (23.2873, 16.0221) (23.2552, 16.0018) (23.2342, 15.9877) (23.2237, 15.9805) knots -1 -1 -1 -1 -1 -1 -0.98571429 -0.97142857 -0.95714286 -0.94285714 -0.92857143 -0.91428571 -0.9 -0.88571429 -0.87142857 -0.85714286 -0.84285714 -0.82857143 -0.81428571 -0.8 -0.78571429 -0.77142857 -0.75714286 -0.74285714 -0.72857143 -0.71428571 -0.7 -0.68571429 -0.67142857 -0.65714286 -0.64285714 -0.62857143 -0.61428571 -0.6 -0.58571429 -0.57142857 -0.55714286 -0.54285714 -0.52857143 -0.51428571 -0.5 -0.48571429 -0.47142857 -0.45714286 -0.44285714 -0.42857143 -0.41428571 -0.4 -0.38571429 -0.37142857 -0.35714286 -0.34285714 -0.32857143 -0.31428571 -0.3 -0.28571429 -0.27142857 -0.25714286 -0.24285714 -0.22857143 -0.21428571 -0.2 -0.18571429 -0.17142857 -0.15714286 -0.14285714 -0.12857143 -0.11428571 -0.1 -0.08571429 -0.07142857 -0.05714286 -0.04285714 -0.02857143 -0.01428571 0 0 0 0 0 0
  line L29 (23.2237, 15.9805) -> (22.9298, 15.7785)
  arc A59 (21.6955, 15.9864) -> (22.9298, 15.7785) centre (22.42, 16.5203) ccw
  arc A60 (21.6955, 15.9864) -> (21.0569, 16.8187) centre (0, 0) ccw
  arc A61 (21.1755, 18.0647) -> (21.0569, 16.8187) centre (21.7601, 17.3803) ccw
  line L30 (21.1755, 18.0647) -> (21.4468, 18.2963)
  spline S30 degree 5 poles (21.4468, 18.2963) (21.4564, 18.3046) (21.4754, 18.3212) (21.5033, 18.3469) (21.5393, 18.3825) (21.5826, 18.4288) (21.6246, 18.4763) (21.6659, 18.5247) (21.7068, 18.5735) (21.7474, 18.6226) (21.7877, 18.6721) (21.8276, 18.7219) (21.867, 18.7722) (21.9058, 18.8232) (21.944, 18.8747) (21.9816, 18.9269) (22.0187, 18.9795) (22.0554, 19.0325) (22.0917, 19.0858) (22.1277, 19.1395) (22.1634, 19.1935) (22.1987, 19.2479) (22.2336, 19.3026) (22.2681, 19.3576) (22.3022, 19.413) (22.336, 19.4688) (22.3694, 19.5249) (22.4024, 19.5813) (22.4351, 19.638) (22.4675, 19.695) (22.4995, 19.7522) (22.5312, 19.8098) (22.5626, 19.8676) (22.5937, 19.9257) (22.6244, 19.9841) (22.6549, 20.0428) (22.685, 20.1017) (22.7148, 20.1609) (22.7443, 20.2203) (22.7735, 20.28) (22.8023, 20.3399) (22.8309, 20.4) (22.8592, 20.4604) (22.8872, 20.5211) (22.9149, 20.5819) (22.9423, 20.643) (22.9694, 20.7043) (22.9962, 20.7659) (23.0228, 20.8276) (23.049, 20.8896) (23.075, 20.9518) (23.1007, 21.0142) (23.1261, 21.0768) (23.1512, 21.1396) (23.176, 21.2027) (23.2006, 21.2659) (23.2249, 21.3293) (23.2489, 21.3929) (23.2726, 21.4567) (23.2961, 21.5207) (23.3193, 21.5849) (23.3422, 21.6493) (23.3649, 21.7139) (23.3872, 21.7786) (23.4094, 21.8436) (23.4312, 21.9087) (23.4528, 21.974) (23.4741, 22.0394) (23.4952, 22.1051) (23.516, 22.1709) (23.5365, 22.2369) (23.5527, 22.2898) (23.5648, 22.3295) (23.5727, 22.3561) (23.5767, 22.3694) knots 0 0 0 0 0 0 0.01428571 0.02857143 0.04285714 0.05714286 0.07142857 0.08571429 0.1 0.11428571 0.12857143 0.14285714 0.15714286 0.17142857 0.18571429 0.2 0.21428571 0.22857143 0.24285714 0.25714286 0.27142857 0.28571429 0.3 0.31428571 0.32857143 0.34285714 0.35714286 0.37142857 0.38571429 0.4 0.41428571 0.42857143 0.44285714 0.45714286 0.47142857 0.48571429 0.5 0.51428571 0.52857143 0.54285714 0.55714286 0.57142857 0.58571429 0.6 0.61428571 0.62857143 0.64285714 0.65714286 0.67142857 0.68571429 0.7 0.71428571 0.72857143 0.74285714 0.75714286 0.77142857 0.78571429 0.8 0.81428571 0.82857143 0.84285714 0.85714286 0.87142857 0.88571429 0.9 0.91428571 0.92857143 0.94285714 0.95714286 0.97142857 0.98571429 1 1 1 1 1 1
  arc A62 (23.5767, 22.3694) -> (22.3694, 23.5767) centre (0, 0) ccw
  spline S31 degree 5 poles (22.3694, 23.5767) (22.3561, 23.5727) (22.3295, 23.5648) (22.2898, 23.5527) (22.2369, 23.5365) (22.1709, 23.516) (22.1051, 23.4952) (22.0394, 23.4741) (21.974, 23.4528) (21.9087, 23.4312) (21.8436, 23.4094) (21.7786, 23.3872) (21.7139, 23.3649) (21.6493, 23.3422) (21.5849, 23.3193) (21.5207, 23.2961) (21.4567, 23.2726) (21.3929, 23.2489) (21.3293, 23.2249) (21.2659, 23.2006) (21.2027, 23.176) (21.1396, 23.1512) (21.0768, 23.1261) (21.0142, 23.1007) (20.9518, 23.075) (20.8896, 23.049) (20.8276, 23.0228) (20.7659, 22.9962) (20.7043, 22.9694) (20.643, 22.9423) (20.5819, 22.9149) (20.5211, 22.8872) (20.4604, 22.8592) (20.4, 22.8309) (20.3399, 22.8023) (20.28, 22.7735) (20.2203, 22.7443) (20.1609, 22.7148) (20.1017, 22.685) (20.0428, 22.6549) (19.9841, 22.6244) (19.9257, 22.5937) (19.8676, 22.5626) (19.8098, 22.5312) (19.7522, 22.4995) (19.695, 22.4675) (19.638, 22.4351) (19.5813, 22.4024) (19.5249, 22.3694) (19.4688, 22.336) (19.413, 22.3022) (19.3576, 22.2681) (19.3026, 22.2336) (19.2479, 22.1987) (19.1935, 22.1634) (19.1395, 22.1277) (19.0858, 22.0917) (19.0325, 22.0554) (18.9795, 22.0187) (18.9269, 21.9816) (18.8747, 21.944) (18.8232, 21.9058) (18.7722, 21.867) (18.7219, 21.8276) (18.6721, 21.7877) (18.6226, 21.7474) (18.5735, 21.7068) (18.5247, 21.6659) (18.4763, 21.6246) (18.4288, 21.5826) (18.3825, 21.5393) (18.3469, 21.5033) (18.3212, 21.4754) (18.3046, 21.4564) (18.2963, 21.4468) knots -1 -1 -1 -1 -1 -1 -0.98571429 -0.97142857 -0.95714286 -0.94285714 -0.92857143 -0.91428571 -0.9 -0.88571429 -0.87142857 -0.85714286 -0.84285714 -0.82857143 -0.81428571 -0.8 -0.78571429 -0.77142857 -0.75714286 -0.74285714 -0.72857143 -0.71428571 -0.7 -0.68571429 -0.67142857 -0.65714286 -0.64285714 -0.62857143 -0.61428571 -0.6 -0.58571429 -0.57142857 -0.55714286 -0.54285714 -0.52857143 -0.51428571 -0.5 -0.48571429 -0.47142857 -0.45714286 -0.44285714 -0.42857143 -0.41428571 -0.4 -0.38571429 -0.37142857 -0.35714286 -0.34285714 -0.32857143 -0.31428571 -0.3 -0.28571429 -0.27142857 -0.25714286 -0.24285714 -0.22857143 -0.21428571 -0.2 -0.18571429 -0.17142857 -0.15714286 -0.14285714 -0.12857143 -0.11428571 -0.1 -0.08571429 -0.07142857 -0.05714286 -0.04285714 -0.02857143 -0.01428571 0 0 0 0 0 0
  line L31 (18.2963, 21.4468) -> (18.0647, 21.1755)
  arc A63 (16.8187, 21.0569) -> (18.0647, 21.1755) centre (17.3803, 21.7601) ccw
  arc A64 (16.8187, 21.0569) -> (15.9864, 21.6955) centre (0, 0) ccw
  arc A65 (15.7785, 22.9298) -> (15.9864, 21.6955) centre (16.5203, 22.42) ccw
  line L32 (15.7785, 22.9298) -> (15.9805, 23.2237)
  spline S32 degree 5 poles (15.9805, 23.2237) (15.9877, 23.2342) (16.0018, 23.2552) (16.0221, 23.2873) (16.0476, 23.3309) (16.0774, 23.3868) (16.1057, 23.4436) (16.1331, 23.501) (16.1599, 23.5588) (16.1864, 23.6167) (16.2126, 23.6749) (16.2383, 23.7333) (16.2633, 23.7922) (16.2876, 23.8514) (16.3111, 23.9111) (16.3339, 23.9712) (16.3562, 24.0316) (16.3779, 24.0923) (16.3992, 24.1533) (16.4201, 24.2144) (16.4405, 24.2758) (16.4606, 24.3375) (16.4801, 24.3993) (16.4992, 24.4614) (16.5178, 24.5238) (16.536, 24.5864) (16.5537, 24.6492) (16.571, 24.7123) (16.5879, 24.7755) (16.6045, 24.8389) (16.6206, 24.9025) (16.6364, 24.9663) (16.6517, 25.0303) (16.6667, 25.0945) (16.6813, 25.1588) (16.6955, 25.2233) (16.7093, 25.288) (16.7228, 25.3529) (16.7359, 25.4179) (16.7486, 25.4831) (16.761, 25.5485) (16.7731, 25.614) (16.7848, 25.6797) (16.7961, 25.7455) (16.8071, 25.8114) (16.8178, 25.8775) (16.8281, 25.9438) (16.838, 26.0102) (16.8477, 26.0767) (16.857, 26.1433) (16.866, 26.2101) (16.8746, 26.2771) (16.883, 26.3441) (16.891, 26.4113) (16.8987, 26.4786) (16.906, 26.546) (16.9131, 26.6136) (16.9198, 26.6812) (16.9262, 26.749) (16.9323, 26.8169) (16.9381, 26.8849) (16.9436, 26.953) (16.9488, 27.0213) (16.9536, 27.0896) (16.9582, 27.158) (16.9624, 27.2266) (16.9664, 27.2952) (16.97, 27.364) (16.9734, 27.4329) (16.9764, 27.5018) (16.9792, 27.5708) (16.9812, 27.6262) (16.9825, 27.6677) (16.9833, 27.6954) (16.9837, 27.7093) knots 0 0 0 0 0 0 0.01428571 0.02857143 0.04285714 0.05714286 0.07142857 0.08571429 0.1 0.11428571 0.12857143 0.14285714 0.15714286 0.17142857 0.18571429 0.2 0.21428571 0.22857143 0.24285714 0.25714286 0.27142857 0.28571429 0.3 0.31428571 0.32857143 0.34285714 0.35714286 0.37142857 0.38571429 0.4 0.41428571 0.42857143 0.44285714 0.45714286 0.47142857 0.48571429 0.5 0.51428571 0.52857143 0.54285714 0.55714286 0.57142857 0.58571429 0.6 0.61428571 0.62857143 0.64285714 0.65714286 0.67142857 0.68571429 0.7 0.71428571 0.72857143 0.74285714 0.75714286 0.77142857 0.78571429 0.8 0.81428571 0.82857143 0.84285714 0.85714286 0.87142857 0.88571429 0.9 0.91428571 0.92857143 0.94285714 0.95714286 0.97142857 0.98571429 1 1 1 1 1 1
  arc A66 (16.9837, 27.7093) -> (15.5051, 28.563) centre (0, 0) ccw
  spline S33 degree 5 poles (15.5051, 28.563) (15.4933, 28.5557) (15.4697, 28.5411) (15.4344, 28.5192) (15.3875, 28.4898) (15.329, 28.4529) (15.2709, 28.4158) (15.2129, 28.3785) (15.1552, 28.3409) (15.0977, 28.3032) (15.0405, 28.2652) (14.9835, 28.2271) (14.9267, 28.1887) (14.8702, 28.1501) (14.814, 28.1113) (14.758, 28.0723) (14.7022, 28.033) (14.6467, 27.9936) (14.5915, 27.9539) (14.5365, 27.9141) (14.4818, 27.874) (14.4274, 27.8337) (14.3732, 27.7931) (14.3193, 27.7524) (14.2657, 27.7114) (14.2123, 27.6703) (14.1592, 27.6289) (14.1064, 27.5873) (14.0539, 27.5454) (14.0017, 27.5034) (13.9498, 27.4611) (13.8982, 27.4186) (13.8469, 27.3759) (13.7958, 27.3329) (13.7451, 27.2897) (13.6947, 27.2463) (13.6446, 27.2027) (13.5949, 27.1588) (13.5454, 27.1147) (13.4963, 27.0704) (13.4475, 27.0258) (13.3991, 26.981) (13.351, 26.936) (13.3033, 26.8907) (13.2559, 26.8451) (13.2089, 26.7993) (13.1622, 26.7533) (13.1159, 26.7071) (13.07, 26.6606) (13.0245, 26.6138) (12.9793, 26.5668) (12.9346, 26.5195) (12.8904, 26.4719) (12.8466, 26.424) (12.8032, 26.3758) (12.7603, 26.3274) (12.7178, 26.2788) (12.6756, 26.2299) (12.6339, 26.1807) (12.5927, 26.1312) (12.5521, 26.0814) (12.5122, 26.0312) (12.473, 25.9805) (12.4346, 25.9294) (12.3968, 25.878) (12.3595, 25.8262) (12.3225, 25.7743) (12.2859, 25.7222) (12.2499, 25.6698) (12.2149, 25.6169) (12.1814, 25.5631) (12.1563, 25.5192) (12.1387, 25.4856) (12.1275, 25.4629) (12.1221, 25.4514) knots -1 -1 -1 -1 -1 -1 -0.98571429 -0.97142857 -0.95714286 -0.94285714 -0.92857143 -0.91428571 -0.9 -0.88571429 -0.87142857 -0.85714286 -0.84285714 -0.82857143 -0.81428571 -0.8 -0.78571429 -0.77142857 -0.75714286 -0.74285714 -0.72857143 -0.71428571 -0.7 -0.68571429 -0.67142857 -0.65714286 -0.64285714 -0.62857143 -0.61428571 -0.6 -0.58571429 -0.57142857 -0.55714286 -0.54285714 -0.52857143 -0.51428571 -0.5 -0.48571429 -0.47142857 -0.45714286 -0.44285714 -0.42857143 -0.41428571 -0.4 -0.38571429 -0.37142857 -0.35714286 -0.34285714 -0.32857143 -0.31428571 -0.3 -0.28571429 -0.27142857 -0.25714286 -0.24285714 -0.22857143 -0.21428571 -0.2 -0.18571429 -0.17142857 -0.15714286 -0.14285714 -0.12857143 -0.11428571 -0.1 -0.08571429 -0.07142857 -0.05714286 -0.04285714 -0.02857143 -0.01428571 0 0 0 0 0 0
  line L33 (12.1221, 25.4514) -> (11.9685, 25.1295)
  arc A67 (10.7957, 24.6924) -> (11.9685, 25.1295) centre (11.1562, 25.517) ccw
  arc A68 (10.7957, 24.6924) -> (9.8265, 25.0938) centre (0, 0) ccw
  arc A69 (9.3062, 26.2322) -> (9.8265, 25.0938) centre (10.1546, 25.9319) ccw
  line L34 (9.3062, 26.2322) -> (9.4253, 26.5685)
  spline S34 degree 5 poles (9.4253, 26.5685) (9.4295, 26.5804) (9.4376, 26.6044) (9.449, 26.6406) (9.4623, 26.6894) (9.4767, 26.7511) (9.4893, 26.8133) (9.5009, 26.8758) (9.5119, 26.9385) (9.5225, 27.0014) (9.5326, 27.0643) (9.5423, 27.1274) (9.5513, 27.1907) (9.5594, 27.2542) (9.5667, 27.318) (9.5732, 27.3819) (9.579, 27.4461) (9.5843, 27.5103) (9.5891, 27.5747) (9.5934, 27.6392) (9.5973, 27.7038) (9.6007, 27.7685) (9.6036, 27.8333) (9.6059, 27.8982) (9.6078, 27.9633) (9.6091, 28.0285) (9.61, 28.0937) (9.6104, 28.1591) (9.6104, 28.2246) (9.6099, 28.2901) (9.609, 28.3557) (9.6077, 28.4214) (9.606, 28.4872) (9.6039, 28.553) (9.6013, 28.619) (9.5983, 28.685) (9.5949, 28.7511) (9.5911, 28.8172) (9.587, 28.8834) (9.5824, 28.9497) (9.5775, 29.016) (9.5721, 29.0824) (9.5664, 29.1489) (9.5604, 29.2154) (9.5539, 29.2819) (9.5471, 29.3485) (9.5399, 29.4152) (9.5324, 29.4819) (9.5245, 29.5487) (9.5162, 29.6154) (9.5076, 29.6823) (9.4986, 29.7492) (9.4893, 29.8161) (9.4797, 29.8831) (9.4697, 29.9501) (9.4594, 30.0171) (9.4487, 30.0842) (9.4377, 30.1513) (9.4263, 30.2184) (9.4146, 30.2855) (9.4026, 30.3527) (9.3903, 30.42) (9.3776, 30.4872) (9.3646, 30.5545) (9.3513, 30.6218) (9.3377, 30.6891) (9.3237, 30.7564) (9.3095, 30.8238) (9.2949, 30.8911) (9.28, 30.9585) (9.2648, 31.0259) (9.2524, 31.0799) (9.2429, 31.1203) (9.2365, 31.1473) (9.2333, 31.1608) knots 0 0 0 0 0 0 0.01428571 0.02857143 0.04285714 0.05714286 0.07142857 0.08571429 0.1 0.11428571 0.12857143 0.14285714 0.15714286 0.17142857 0.18571429 0.2 0.21428571 0.22857143 0.24285714 0.25714286 0.27142857 0.28571429 0.3 0.31428571 0.32857143 0.34285714 0.35714286 0.37142857 0.38571429 0.4 0.41428571 0.42857143 0.44285714 0.45714286 0.47142857 0.48571429 0.5 0.51428571 0.52857143 0.54285714 0.55714286 0.57142857 0.58571429 0.6 0.61428571 0.62857143 0.64285714 0.65714286 0.67142857 0.68571429 0.7 0.71428571 0.72857143 0.74285714 0.75714286 0.77142857 0.78571429 0.8 0.81428571 0.82857143 0.84285714 0.85714286 0.87142857 0.88571429 0.9 0.91428571 0.92857143 0.94285714 0.95714286 0.97142857 0.98571429 1 1 1 1 1 1
  arc A70 (9.2333, 31.1608) -> (7.5841, 31.6027) centre (0, 0) ccw
  spline S35 degree 5 poles (7.5841, 31.6027) (7.5746, 31.5926) (7.5556, 31.5725) (7.5272, 31.5421) (7.4894, 31.5016) (7.4426, 31.4509) (7.396, 31.4) (7.3496, 31.3489) (7.3036, 31.2977) (7.2579, 31.2464) (7.2124, 31.1949) (7.1672, 31.1433) (7.1223, 31.0915) (7.0777, 31.0396) (7.0335, 30.9876) (6.9895, 30.9354) (6.9458, 30.883) (6.9024, 30.8306) (6.8593, 30.778) (6.8165, 30.7252) (6.774, 30.6724) (6.7319, 30.6193) (6.69, 30.5662) (6.6485, 30.5129) (6.6073, 30.4594) (6.5664, 30.4058) (6.5259, 30.3521) (6.4857, 30.2983) (6.4458, 30.2443) (6.4062, 30.1901) (6.367, 30.1358) (6.3282, 30.0814) (6.2896, 30.0269) (6.2515, 29.9722) (6.2137, 29.9173) (6.1762, 29.8624) (6.1391, 29.8073) (6.1024, 29.752) (6.0661, 29.6966) (6.0301, 29.6411) (5.9945, 29.5854) (5.9593, 29.5296) (5.9245, 29.4736) (5.8902, 29.4175) (5.8562, 29.3613) (5.8226, 29.3049) (5.7895, 29.2484) (5.7567, 29.1917) (5.7244, 29.1349) (5.6925, 29.0779) (5.6611, 29.0208) (5.6301, 28.9636) (5.5997, 28.9061) (5.5698, 28.8486) (5.5404, 28.7908) (5.5114, 28.7329) (5.483, 28.6749) (5.4549, 28.6168) (5.4274, 28.5585) (5.4004, 28.5) (5.374, 28.4414) (5.3485, 28.3826) (5.3237, 28.3235) (5.2998, 28.2642) (5.2766, 28.2047) (5.254, 28.1451) (5.2318, 28.0854) (5.2099, 28.0256) (5.1887, 27.9656) (5.1685, 27.9054) (5.1501, 27.8448) (5.1373, 27.7959) (5.1289, 27.7589) (5.124, 27.7341) (5.1217, 27.7216) knots -1 -1 -1 -1 -1 -1 -0.98571429 -0.97142857 -0.95714286 -0.94285714 -0.92857143 -0.91428571 -0.9 -0.88571429 -0.87142857 -0.85714286 -0.84285714 -0.82857143 -0.81428571 -0.8 -0.78571429 -0.77142857 -0.75714286 -0.74285714 -0.72857143 -0.71428571 -0.7 -0.68571429 -0.67142857 -0.65714286 -0.64285714 -0.62857143 -0.61428571 -0.6 -0.58571429 -0.57142857 -0.55714286 -0.54285714 -0.52857143 -0.51428571 -0.5 -0.48571429 -0.47142857 -0.45714286 -0.44285714 -0.42857143 -0.41428571 -0.4 -0.38571429 -0.37142857 -0.35714286 -0.34285714 -0.32857143 -0.31428571 -0.3 -0.28571429 -0.27142857 -0.25714286 -0.24285714 -0.22857143 -0.21428571 -0.2 -0.18571429 -0.17142857 -0.15714286 -0.14285714 -0.12857143 -0.11428571 -0.1 -0.08571429 -0.07142857 -0.05714286 -0.04285714 -0.02857143 -0.01428571 0 0 0 0 0 0
  line L35 (5.1217, 27.7216) -> (5.0567, 27.3709)
  arc A71 (4.037, 26.6451) -> (5.0567, 27.3709) centre (4.1718, 27.535) ccw
  arc A72 (4.037, 26.6451) -> (2.9969, 26.782) centre (0, 0) ccw
  arc A73 (2.1997, 27.747) -> (2.9969, 26.782) centre (3.097, 27.6765) ccw
  line L36 (2.1997, 27.747) -> (2.2277, 28.1026)
  spline S36 degree 5 poles (2.2277, 28.1026) (2.2287, 28.1152) (2.2303, 28.1405) (2.2319, 28.1784) (2.2322, 28.229) (2.2301, 28.2923) (2.2262, 28.3557) (2.2212, 28.419) (2.2155, 28.4825) (2.2095, 28.5459) (2.2031, 28.6093) (2.1961, 28.6728) (2.1883, 28.7363) (2.1797, 28.7997) (2.1703, 28.8632) (2.16, 28.9266) (2.1491, 28.9901) (2.1375, 29.0535) (2.1255, 29.117) (2.113, 29.1804) (2.1, 29.2438) (2.0865, 29.3071) (2.0726, 29.3705) (2.058, 29.4338) (2.043, 29.4972) (2.0274, 29.5604) (2.0113, 29.6237) (1.9948, 29.687) (1.9778, 29.7502) (1.9604, 29.8134) (1.9426, 29.8765) (1.9244, 29.9396) (1.9057, 30.0027) (1.8865, 30.0658) (1.867, 30.1288) (1.847, 30.1918) (1.8267, 30.2547) (1.8059, 30.3177) (1.7847, 30.3805) (1.7632, 30.4434) (1.7412, 30.5062) (1.7189, 30.5689) (1.6962, 30.6316) (1.6731, 30.6943) (1.6497, 30.7569) (1.6258, 30.8195) (1.6016, 30.882) (1.5771, 30.9445) (1.5522, 31.0069) (1.5269, 31.0693) (1.5013, 31.1316) (1.4753, 31.1939) (1.449, 31.2562) (1.4224, 31.3183) (1.3954, 31.3805) (1.368, 31.4425) (1.3404, 31.5046) (1.3124, 31.5665) (1.284, 31.6284) (1.2554, 31.6903) (1.2264, 31.7521) (1.1971, 31.8138) (1.1674, 31.8755) (1.1375, 31.9371) (1.1072, 31.9986) (1.0766, 32.0601) (1.0457, 32.1216) (1.0145, 32.1829) (0.983, 32.2442) (0.9511, 32.3055) (0.919, 32.3666) (0.893, 32.4155) (0.8734, 32.4522) (0.8603, 32.4766) (0.8537, 32.4888) knots 0 0 0 0 0 0 0.01428571 0.02857143 0.04285714 0.05714286 0.07142857 0.08571429 0.1 0.11428571 0.12857143 0.14285714 0.15714286 0.17142857 0.18571429 0.2 0.21428571 0.22857143 0.24285714 0.25714286 0.27142857 0.28571429 0.3 0.31428571 0.32857143 0.34285714 0.35714286 0.37142857 0.38571429 0.4 0.41428571 0.42857143 0.44285714 0.45714286 0.47142857 0.48571429 0.5 0.51428571 0.52857143 0.54285714 0.55714286 0.57142857 0.58571429 0.6 0.61428571 0.62857143 0.64285714 0.65714286 0.67142857 0.68571429 0.7 0.71428571 0.72857143 0.74285714 0.75714286 0.77142857 0.78571429 0.8 0.81428571 0.82857143 0.84285714 0.85714286 0.87142857 0.88571429 0.9 0.91428571 0.92857143 0.94285714 0.95714286 0.97142857 0.98571429 1 1 1 1 1 1
  arc A74 (0.8537, 32.4888) -> (-0.8537, 32.4888) centre (0, 0) ccw